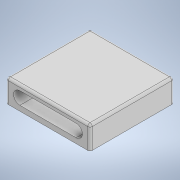
# Autodesk Inventor part: T5 SSD
Saved by Autodesk Inventor 2021 (Build 250183000, 183)
## iProperties
Created: 2022-08-23
Part Number: T5 SSD
Material: Generic
Document SubType Name: Modeling
Designer: cmzgt
Density: 1 g/cm^3
Appearance: Default
Author: cmzgt
Autodesk Inventor part; units mm, degrees
ref_plane "YZ Plane" through (0, 0, 0) normal (1, 0, 0) x (0, 1, 0)
ref_plane "XZ Plane" through (0, 0, 0) normal (0, 1, 0) x (-1, 0, 0)
ref_plane "XY Plane" through (0, 0, 0) normal (0, 0, 1) x (1, 0, 0)
sketch "Sketch1" plane through (0, 0, 0) normal (0, 0, 1) x (1, 0, 0)
  line L0 (34.925, -9.525) -> (-34.925, -9.525)
  line L1 (-34.925, -9.525) -> (-34.925, 9.525)
  line L2 (-34.925, 9.525) -> (34.925, 9.525)
  line L3 (34.925, 9.525) -> (34.925, -9.525)
  line L4 (34.925, -9.525) -> (-34.925, 9.525) construction
  line L5 (-34.925, -9.525) -> (34.925, 9.525) construction
  point P0 (0, 0)
  dimension "d0" = 69.85
  dimension "d1" = 19.05
  constraints: 12 end point, 2 midpoint, 2 parallel, 1 horizontal, 1 perpendicular
  measures "d0" distance of L1.end L2.end
  measures "d1" distance of L0.end L1.end
extrude "Extrusion1" add sketch "Sketch1" along normal blind 69.85
fillet "Fillet1" radius 1.905 8 edges at (34.925, 9.525, 34.925) (-34.925, 9.525, 34.925) (0, 9.525, 0) (0, 9.525, 69.85) (34.925, 0, 69.85) (-34.925, 0, 69.85) (34.925, 0, 0) (-34.925, 0, 0)
sketch "Sketch2" plane through (0, 0, 69.85) normal (0, 0, 1) x (1, 0, 0)
  line L0 (23.4, -5.25) -> (-23.4, -5.25)
  line L1 (-28.65, 0) -> (-28.65, 0)
  line L2 (-23.4, 5.25) -> (23.4, 5.25)
  line L3 (28.65, 0) -> (28.65, 0)
  line L4 (28.65, -5.25) -> (-28.65, 5.25) construction
  line L5 (-28.65, -5.25) -> (28.65, 5.25) construction
  arc A0 (-23.4, 5.25) -> (-28.65, 0) centre (-23.4, 0) ccw
  arc A1 (-28.65, 0) -> (-23.4, -5.25) centre (-23.4, 0) ccw
  arc A2 (28.65, 0) -> (23.4, 5.25) centre (23.4, 0) ccw
  arc A3 (23.4, -5.25) -> (28.65, 0) centre (23.4, 0) ccw
  point P0 (0, 0)
  point P1 (28.65, 0)
  dimension "d5" = 57.3
  dimension "d6" = 10.5
  dimension "d9" = 5.25
  constraints: 12 end point, 8 point on circle, 8 point on line, 8 tangent, 4 centre point, 3 equal radius, 2 midpoint, 2 parallel, 1 horizontal, 1 perpendicular
  measures "d5" distance of L4.end L5.end
  measures "d6" distance of L5.start L4.end
  measures "d9" radius of A0
extrude "Extrusion2" cut sketch "Sketch2" against normal blind 66.04
body "Solid1"
